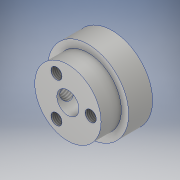
# Autodesk Inventor part: 6mm Mounting Hub, thin
Saved by Autodesk Inventor 2017 (Build 210142000, 142)
## iProperties
Created: 2016-03-07
Part Number: 6mm Mounting Hub, thin
Material: Aluminum 6061
Description: STEP AP214
Document SubType Name: Modeling
Designer: Zach
Density: 2.7 g/cm^3
Appearance: Aluminum - Flat
Mass: 8.84704 g
Surface Area: 19.8706 cm^2
Volume: 3.27668 cm^3
Sending System: SolidWorks 2015
Preprocessor: SwSTEP 2.0
Title: hub02-6mm.step
Revision Number: ANY
Autodesk Inventor part; units mm, degrees
ref_plane "YZ Plane" through (0, 0, 0) normal (1, 0, 0) x (0, 1, 0)
ref_plane "XZ Plane" through (0, 0, 0) normal (0, 1, 0) x (-1, 0, 0)
ref_plane "XY Plane" through (0, 0, 0) normal (0, 0, 1) x (1, 0, 0)
sketch "Sketch3" plane through (0, 0, 0) normal (0, 0, 1) x (1, 0, 0)
  circle A0 centre (0, 0) radius 11
  circle A1 centre (0, 0) radius 3
  circle A2 centre (6.2, 0) radius 1.5
  circle A3 centre (3.1, 5.3694) radius 1.5
  circle A4 centre (-3.1, 5.3694) radius 1.5
  circle A5 centre (-6.2, 0) radius 1.5
  circle A6 centre (-3.1, -5.3694) radius 1.5
  circle A7 centre (3.1, -5.3694) radius 1.5
  dimension "d0" = 22
  dimension "d1" = 6
  dimension "d4" = 3
  dimension "d5" = 6.2
  dimension "d12" = 360
  constraints: 8 centre point, 2 coincident, 1 horizontal alignment, 13 other
  measures "d0" diameter of A0
  measures "d1" diameter of A1
  measures "d4" diameter of A2
  measures "d5" distance of point (0, 0) A2.centre
extrude "Extrusion1" add sketch "Sketch3" along normal blind 6.5 contours A0 | A3 | A5 | A7
sketch "Sketch6" plane through (0, 0, 6.5) normal (0, 0, 1) x (1, 0, 0)
  circle A0 centre (0, 0) radius 3 projected
  circle A1 centre (-3.1, -5.3694) radius 1.5 projected
  circle A2 centre (-3.1, 5.3694) radius 1.5 projected
  circle A3 centre (6.2, 0) radius 1.5 projected
  circle A4 centre (0, 0) radius 11 projected
  circle A5 centre (0, 0) radius 9
  dimension "d27" = 18
  constraints: 1 centre point, 1 coincident
  measures "d27" diameter of A5
extrude "Extrusion4" add sketch "Sketch6" along normal blind 5.5 contours A5
sketch "Sketch7" plane through (0, 0, 0) normal (1, 0, 0) x (0, 1, 0)
  circle A0 centre (0, 3.25) radius 2
  circle A1 centre (0, 9.25) radius 2
  line L0 (11, 0) -> (11, 6.5) projected
  line L1 (9, 6.5) -> (9, 12) projected
  point P0 (0, 0)
  point P1 (11, 3.25)
  point P2 (9, 9.25)
  dimension "d30" = 4
  dimension "d31" = 4
  constraints: 2 centre point, 2 horizontal alignment, 2 midpoint, 2 vertical alignment
  measures "d30" diameter of A0
  measures "d31" diameter of A1
extrude "Extrusion5" cut sketch "Sketch7" against normal through all
thread "Thread5" size "M4x0.7" class "6H" standard "ANSI Metric M Profile" full length
thread "Thread6" size "M4x0.7" class "6H" standard "ANSI Metric M Profile" full length
thread "Thread7" size "M3x0.5" class "6H" standard "ANSI Metric M Profile" full length
thread "Thread8" size "M3x0.5" class "6H" standard "ANSI Metric M Profile" full length
thread "Thread9" size "M3x0.5" class "6H" standard "ANSI Metric M Profile" full length
body "Solid2"
